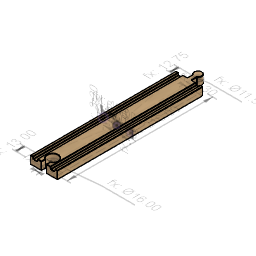
wooden_train_parameter_list_autodesk_fusion_360_example v1 (Autodesk Fusion 360 design; units mm, degrees)
Autodesk Fusion 360 part; units mm, degrees
note: some values were not read from the file. Set by a fixed rule: which sketch regions a step uses.
sketch "Skizze1" plane through (0, 0, 0) normal (0, 1, 0) x (1, 0, 0)
  line L0 (20, 6) -> (-20, 6)
  line L1 (-20, 6) -> (-20, -6)
  line L2 (-20, -6) -> (20, -6) construction
  line L3 (20, -6) -> (20, 6)
  line L4 (20, 6) -> (-20, -6) construction
  line L5 (-20, 6) -> (20, -6) construction
  line L6 (-16.25, -6) -> (-15.75, -2.8)
  line L7 (-15.75, -2.8) -> (-10.25, -2.8)
  line L8 (-10.25, -2.8) -> (-9.75, -6)
  line L9 (-13, -2.8) -> (-13, -6)
  line L10 (0, 6) -> (0, -6) construction
  line L11 (-20, -6) -> (-16.25, -6)
  line L12 (-9.75, -6) -> (0, -6)
  line L13 (20, -6) -> (16.25, -6)
  line L14 (16.25, -6) -> (15.75, -2.8)
  line L15 (15.75, -2.8) -> (10.25, -2.8)
  line L16 (10.25, -2.8) -> (9.75, -6)
  line L17 (9.75, -6) -> (0, -6)
  dimension "d28" = 40
  dimension "d29" = 12
  dimension "d30" = 6.5
  dimension "d31" = 5.5
  dimension "d33" = 3.2
  dimension "d34" = 13
  constraint horizontal L0
  constraint perpendicular L0 L1
  constraint parallel L0 L2
  constraint parallel L1 L3
  constraint coincident L4 origin
  constraint coincident L5 origin
  constraint coincident L2 L6.start
  constraint parallel L2 L7
  constraint coincident L2 L8.end
  constraint midpoint L7 L9.start
  constraint coincident L2 L9.end
  constraint perpendicular L2 L9
  constraint symmetric L6 L8 L9
  constraint midpoint L0 L10.start
  constraint midpoint L2 L10.end
  constraint perpendicular L10 L12
  constraint symmetric L1.end L10 L2.end
  constraint symmetric L6.start L10 L13.end
  constraint symmetric L6.end L10 L14.end
  constraint symmetric L7.end L10 L15.end
  constraint symmetric L8.end L10 L16.end
  constraint symmetric L12.end L10 L17.end
  measures "d28" distance of L0.start L0.end
  measures "d29" distance of L0.start L2.end
  measures "d30" distance of L6.start L8.end
  measures "d31" distance of L6.end L7.end
  measures "d33" vertical distance of L1.end L6.end
  measures "d34" distance of L9.end L10.end
sketch "Skizze2" plane through (0, 0, 0) normal (0, 0, 1) x (1, 0, 0)
  line L0 (20, 108) -> (-20, 108) construction
  line L1 (-20, 108) -> (-20, -108) construction
  line L2 (-20, -108) -> (20, -108) construction
  line L3 (20, -108) -> (20, 108) construction
  line L4 (20, 108) -> (-20, -108) construction
  line L5 (-20, 108) -> (20, -108) construction
  line L6 (0, 108) -> (0, -108)
  circle A0 centre (0, -95) radius 8
  circle A1 centre (0, 120.75) radius 5.75
  line L7 (3.15, 115.9396) -> (3.15, 108)
  line L8 (-3.15, 115.9396) -> (-3.15, 108)
  line L9 (3.65, -102.1188) -> (3.65, -108)
  line L10 (-3.65, -102.1188) -> (-3.65, -108)
  line L11 (-3.65, -108) -> (3.65, -108)
  line L12 (-3.15, 108) -> (3.15, 108)
  point P0 (20, 0)
  point P1 (-20, 0)
  dimension "d35" = 216
  dimension "d36" = 16
  dimension "d37" = 13
  dimension "d38" = 7.3
  dimension "d39" = 11.5
  dimension "d40" = 12.75
  dimension "d41" = 6.3
  constraint horizontal L0
  constraint perpendicular L0 L1
  constraint parallel L0 L2
  constraint parallel L1 L3
  constraint coincident L4 origin
  constraint coincident L5 origin
  constraint midpoint L0 L6.start
  constraint midpoint L2 L6.end
  constraint coincident L3 P0
  constraint coincident L6 A0.centre
  constraint vertical L6.start A1.centre
  constraint coincident A1 L7.start
  constraint coincident L0 L7.end
  constraint perpendicular L0 L7
  constraint coincident A1 L8.start
  constraint coincident L0 L8.end
  constraint perpendicular L0 L8
  constraint coincident A0 L9.start
  constraint coincident L2 L9.end
  constraint perpendicular L2 L9
  constraint coincident A0 L10.start
  constraint coincident L2 L10.end
  constraint perpendicular L2 L10
  constraint symmetric L6 L7 L8
  measures "d35" distance of L0.start L2.end
  measures "d36" diameter of A0
  measures "d37" vertical distance of L1.end A0.centre
  measures "d38" distance of L9.end L10.end
  measures "d39" diameter of A1
  measures "d40" vertical distance of L0.end A1.centre
  measures "d41" distance of L7.end L8.end
extrude "Extrusion1" add sketch "Skizze1" along normal mid plane 216 in component "long track"
extrude "Extrusion2" cut sketch "Skizze2" along normal mid plane 12 contours L6 A0 | L6 A0 | L6 A0 L9 L11 | L6 A0 L10 L11 in component "long track"
extrude "Extrusion3" add sketch "Skizze2" along normal mid plane 12 contours A1 | A1 L7 L8 L12 in component "long track"
fillet "Abrundung1" radius 0.5 60 edges at (3.65, -105.0594, 6) (20, 0, 6) (6.7, -108, 6) (-16.25, 0, 6) (-10.25, 0, 2.8) (16.25, 0, 6) (15.75, 0, 2.8) (10.25, 0, 2.8) (-20, 0, -6) (-9.75, 0, 6) (20, 0, -6) (-20, 0, 6) (9.75, 0, 6) (-15.75, 0, 2.8) (0, -87, 6) (-13, 108, 2.8) (3.65, -105.0594, -6) (-16, 108, 4.4) (-3.65, -105.0594, -6) (-10, 108, 4.4) (11.825, -108, -6) (20, 108, 0) (-11.575, 108, -6) (-3.15, 111.9698, -6) (-18.125, 108, 6) (16, 108, 4.4) (-3.15, 111.9698, 6) (10, -108, 4.4) (3.15, 111.9698, 6) (3.15, 108, 0) (3.65, -102.1188, 0) (11.575, 108, -6) (-3.65, -105.0594, 6) (10, 108, 4.4) (-3.65, -102.1188, 0) (-10, -108, 4.4) (13, 108, 2.8) (-13, -108, 2.8) (-11.825, -108, -6) (-20, -108, 0) (-3.15, 115.9396, 0) (13, -108, 2.8) (18.125, -108, 6) (3.65, -108, 0) (-3.15, 108, 0) (16, -108, 4.4) (-20, 108, 0) (18.125, 108, 6) (20, -108, 0) (-3.65, -108, 0) (6.45, 108, 6) (-16, -108, 4.4) (3.15, 111.9698, -6) (-18.125, -108, 6) (0, 126.5, -6) (0, -87, -6) (0, 126.5, 6) (-6.7, -108, 6) (3.15, 115.9396, 0) (-6.45, 108, 6) 22 faces at (-10.0833, -36, 3.8667) (-16.0833, -36, 4.9333) (10.0833, -36, 3.8667) (-3.65, -104.0792, -2) (20, -36, 2) (13.9167, -36, 2.8) (3.65, -104.0792, -2) (-20, 36, 2) (11.1333, 108, -3.0667) (-11.3, -108, -3.0667) (16.0833, -36, 4.9333) (-3.15, 110.6465, 2) (11.3, -108, -3.0667) (-13.9167, -36, 2.8) (18.75, -36, 6) (-17.5, 36, 6) (8.1105, 42.9708, -6) (4.3, 43, 6) (-6.6798, -90.5976, 2) (5.6, 122.0546, -2) (3.15, 113.2931, -2) (-11.1333, 108, -3.0667) in component "long track"
component "long track" placed x (1, 0, 0) y (0, 1, 0) z (0, 0, 1) at (0, 0, 0)
equation "track_height = 12 mm"
equation "track_width = 40 mm"
equation "groove_distance_cc = 26 mm"
equation "groove_wide_top = 6.5 mm"
equation "groove_wide_bottom = 5.5 mm"
equation "groove_deep = 3.2 mm"
equation "groove_spacing_double_track_cc = 46 mm" comment "Groove spacing double track center-center"
equation "hole_diameter = 16 mm"
equation "hole_distance = 5 mm"
equation "hole_center_track_end = hole_diameter / 2 + hole_distance"
equation "hole_web_width = 7.3 mm"
equation "spigot_diameter = 11.5 mm"
equation "spigot_distance = 7 mm"
equation "spigot_center_track_end = spigot_diameter / 2 + spigot_distance"
equation "spigot_web_width = 6.3 mm"
equation "long_track_length = 216 mm" comment "d standard track"
equation "middle_track_length = long_track_length * 2 / 3" comment "a b middle track"
equation "short_track_length = long_track_length / 2" comment "A1 B1 C1 short track"
equation "mini_track_length = long_track_length / 4" comment "A2 Bs mini track"
equation "A2_track_length = 72 mm" comment "A2 track = 1/2 A"
equation "long_curve_inner_radius = 182 mm"
equation "long_curve_angle = 45 °"
equation "short_curve_inner_radius = 91 mm"
equation "short_curve_angle = 45 °"
equation "switching_track_lenght = middle_track_length" comment "= middle track"
equation "mechanical_switches_length = long_track_length * 2 / 3"
equation "fillet = 0.5 mm"
equation "d28 = track_width"
equation "d29 = track_height"
equation "d30 = groove_wide_top"
equation "d31 = groove_wide_bottom"
equation "d33 = groove_deep"
equation "d34 = groove_distance_cc / 2"
equation "d35 = long_track_length"
equation "d36 = hole_diameter"
equation "d37 = hole_center_track_end"
equation "d38 = hole_web_width"
equation "d39 = spigot_diameter"
equation "d40 = spigot_center_track_end"
equation "d41 = spigot_web_width"
equation "d42 = long_track_length"
equation "d44 = track_height"
equation "d46 = track_height"
equation "d49 = fillet"
